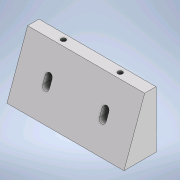
# Autodesk Inventor part: Motorhalterung_BT2.1
Saved by Autodesk Inventor 2020.1 (Build 241239000, 239)
## iProperties
Created: 2020-08-18
Part Number: Motorhalterung_BT2.1
Material: Generisch
Document SubType Name: Modeling
Designer: s5chfeis
Density: 1 g/cm^3
Appearance: Vorgabe
Author: s5chfeis
Autodesk Inventor part; units mm, degrees
ref_plane "YZ Plane" through (0, 0, 0) normal (1, 0, 0) x (0, 1, 0)
ref_plane "XZ Plane" through (0, 0, 0) normal (0, 1, 0) x (-1, 0, 0)
ref_plane "XY Plane" through (0, 0, 0) normal (0, 0, 1) x (1, 0, 0)
sketch "Skizze1" plane through (0, 0, 0) normal (0, 1, 0) x (-1, 0, 0)
  line L0 (0, 0) -> (-206, 0)
  line L1 (-206, 0) -> (-206, -20)
  line L2 (-206, -20) -> (0, -20)
  line L3 (0, -20) -> (0, 0)
  dimension "d0" = 206
  dimension "d1" = 20
  constraints: 8 end point, 2 parallel, 1 horizontal, 1 perpendicular
  measures "d0" distance of L2.end L1.end
  measures "d1" distance of L1.end L0.end
extrude "Extrusion1" add sketch "Skizze1" against normal blind 100
sketch "Skizze2" plane through (0, 0, 0) normal (0, 1, 0) x (1, 0, 0)
  line L0 (0, 0) -> (0, 10) construction
  line L1 (0, 10) -> (206, 10) construction
  line L2 (0, 10) -> (103, 10) construction
  line L3 (103, 10) -> (53, 10) construction
  line L4 (53, 10) -> (153, 10) construction
  dimension "d4" = 10
  dimension "d5" = 206
  dimension "d6" = 90
  dimension "d7" = 103
  dimension "d8" = 50
  dimension "d9" = 100
  constraints: 10 end point, 2 coincident, 2 point on line, 1 midpoint, 1 perpendicular, 1 vertical
  measures "d4" distance of L0.start L0.end
  measures "d5" distance of L0.end L1.end
  measures "d6" angle of L0 L1
  measures "d7" distance of L0.end L2.end
  measures "d8" distance of L2.end L3.end
  measures "d9" distance of L3.end L4.end
hole "Bohrung1" at (153, 0, -10) at (53, 0, -10) direction (0, -1, 0) diameter 8.376 depth 27.3 tip angle 118 thread size "M10x1.5" class "6H" standard "ISO Metric profile"
sketch "Skizze3" plane through (206, 0, 0) normal (1, 0, 0) x (0, 0, -1)
  line L0 (0, 0) -> (-41.0424, -112.7631)
  line L1 (0, 0) -> (120, 0) construction
  line L2 (0, 0) -> (0, -100) projected
  line L3 (0, -100) -> (-50, -100)
  line L4 (0, -100) -> (50, -100) construction
  point P0 (-36.397, -100)
  dimension "d17" = 120
  dimension "d18" = 110
  dimension "d19" = 50
  dimension "d20" = 180
  constraints: 8 end point, 3 horizontal, 2 equal length
  measures "d17" distance of L0.start L0.end
  measures "d18" angle of L0 L1
  measures "d19" distance of L2.end L3.end
  measures "d20" angle of L3 L4
extrude "Extrusion2" add sketch "Skizze3" against normal blind 206
sketch "Skizze4" plane through (206, 0, -20) normal (0, 0, -1) x (-1, 0, 0)
  line L0 (206, 0) -> (103, 0) construction
  line L1 (206, 0) -> (309, 0) construction
  line L2 (103, 0) -> (153, 0) construction
  line L3 (0, 0) -> (206, 0) construction
  line L4 (153, 0) -> (53, 0) construction
  line L5 (53, 0) -> (53, -50) construction
  line L6 (53, 0) -> (103, 0) construction
  line L7 (153, 0) -> (153, -50) construction
  line L8 (153, 0) -> (203, 0) construction
  line L9 (53, -50) -> (59, -50)
  line L10 (59, -50) -> (59, -44)
  arc A0 (59, -44) -> (47, -44) centre (53, -44) ccw
  line L11 (53, -44) -> (47, -44) construction
  line L12 (53, -44) -> (59, -44) construction
  line L13 (47, -44) -> (47, -50)
  line L14 (47, -50) -> (59, -50) construction
  line L15 (53, -100) -> (53, -50) construction
  line L16 (59, -50) -> (59, -56)
  arc A1 (47, -56) -> (59, -56) centre (53, -56) ccw
  line L17 (53, -56) -> (47, -56) construction
  line L18 (53, -56) -> (59, -56) construction
  line L19 (47, -56) -> (47, -50)
  line L20 (103, 0) -> (103, -100) construction
  line L21 (103, 0) -> (203, 0) construction
  line L22 (153, -50) -> (147, -50)
  line L23 (147, -50) -> (147, -44)
  arc A2 (159, -44) -> (147, -44) centre (153, -44) ccw
  line L24 (153, -44) -> (159, -44) construction
  line L25 (153, -44) -> (147, -44) construction
  line L26 (159, -44) -> (159, -50)
  line L27 (159, -50) -> (147, -50) construction
  line L28 (147, -50) -> (147, -56)
  line L29 (153, -56) -> (147, -56) construction
  line L30 (153, -56) -> (159, -56) construction
  line L31 (159, -56) -> (159, -50)
  arc A3 (147, -56) -> (159, -56) centre (153, -56) ccw
  dimension "d23" = 103
  dimension "d24" = 180
  dimension "d25" = 50
  dimension "d26" = 100
  dimension "d27" = 0
  dimension "d28" = 50
  dimension "d29" = 90
  dimension "d30" = 50
  dimension "d31" = 90
  dimension "d32" = 6
  dimension "d33" = 6
  dimension "d34" = 180
  dimension "d35" = 100
  dimension "d36" = 90
  constraints: 62 end point, 15 symmetric about line, 8 point on circle, 7 horizontal, 4 centre point, 4 equal length, 3 perpendicular, 3 point on line, 2 vertical, 1 collinear, 3 other
  measures "d23" distance of L0.start L0.end
  measures "d24" angle of L0 L1
  measures "d25" distance of L0.end L2.end
  measures "d26" distance of L2.end L4.end
  measures "d27" distance between parallel lines of L4 L2
  measures "d28" distance of L4.end L5.end
  measures "d29" angle of L5 L6
  measures "d30" distance of L2.end L7.end
  measures "d31" angle of L7 L8
  measures "d32" distance of L5.end L9.end
  measures "d33" distance of L9.end L10.end
  measures "d34" angle of L12 L11
  measures "d35" distance of L6.end L20.end
  measures "d36" angle of L20 L21
extrude "Extrusion3" cut sketch "Skizze4" against normal blind 100
sketch "Skizze5" plane through (206, 0, -20) normal (0, 0, -1) x (-1, 0, 0)
  line L0 (206, 0) -> (0, 0) projected
  line L1 (103, 0) -> (103, -100)
  line L2 (206, -100) -> (0, -100) projected
  line L3 (0, 0) -> (0, -100) projected
  line L4 (0, -50) -> (206, -50)
  line L5 (206, 0) -> (206, -100) projected
  line L6 (103, -50) -> (68, -50)
  line L7 (68, -50) -> (68, -30)
  line L8 (68, -30) -> (103, -30)
  line L9 (103, -30) -> (103, -50)
  line L10 (103, -50) -> (138, -50)
  line L11 (138, -50) -> (138, -30)
  line L12 (138, -30) -> (103, -30)
  line L13 (68, -50) -> (68, -70)
  line L14 (68, -70) -> (103, -70)
  line L15 (103, -70) -> (103, -50)
  line L16 (138, -50) -> (138, -70)
  line L17 (138, -70) -> (103, -70)
  dimension "d39" = 35
  dimension "d40" = 20
  constraints: 28 end point, 5 midpoint, 5 symmetric about line, 2 parallel, 1 horizontal, 1 perpendicular
  measures "d39" distance of L7.end L8.end
  measures "d40" distance of L6.end L7.end
extrude "Extrusion4" add sketch "Skizze5" along normal blind 30 contours L12 L11 L4 L1 | L1 L4 L7 L8 | L16 L17 L1 L4 | L1 L14 L13 L4
sketch "Skizze6" plane through (68, -30, -20) normal (0, 1, 0) x (1, 0, 0)
  line L0 (70, 30) -> (0, 30) projected
  circle A0 centre (35, 30) radius 17.5
  point P0 (-68, -20)
  dimension "d43" = 35
  constraints: 1 centre point, 1 midpoint
  measures "d43" diameter of A0
extrude "Extrusion5" cut sketch "Skizze6" against normal blind 40
sketch "Skizze7" plane through (68, -30, -20) normal (0, 1, 0) x (1, 0, 0)
  arc A0 (17.5, 30) -> (52.5, 30) centre (35, 30) ccw projected
  line L0 (35, 12.5) -> (35, 13.5)
  line L1 (35, 12.5) -> (36, 12.5) construction
  line L2 (35, 13.5) -> (45, 13.5)
  line L3 (45, 13.5) -> (25, 13.5)
  point P0 (-68, -20)
  point P1 (35, 13.5)
  point P2 (29.169, 13.5)
  point P3 (40.831, 13.5)
  dimension "d46" = 1
  dimension "d47" = 90
  dimension "d48" = 10
  dimension "d49" = 90
  dimension "d50" = 20
  dimension "d51" = 0
  constraints: 8 end point, 2 perpendicular, 1 collinear, 1 horizontal, 1 point on circle, 1 vertical
  measures "d46" distance of L0.start L0.end
  measures "d47" angle of L1 L0
  measures "d48" distance of L0.end L2.end
  measures "d49" angle of L0 L2
  measures "d50" distance of L2.end L3.end
  measures "d51" distance between parallel lines of L3 L2
extrude "Extrusion6" add sketch "Skizze7" against normal blind 40
sketch "Skizze8" plane through (206, 0, -50) normal (0, 0, -1) x (-1, 0, 0)
  line L0 (68, -30) -> (138, -30) construction
  line L1 (85.5, -70) -> (85.5, -30) construction
  line L2 (68, -30) -> (85.5, -70) construction
  line L3 (138, -70) -> (68, -70) construction
  line L4 (68, -70) -> (85.5, -30) construction
  line L5 (103, -30) -> (103, -70) construction
  line L6 (120.5, -70) -> (120.5, -30) construction
  line L7 (138, -30) -> (120.5, -70) construction
  line L8 (138, -70) -> (120.5, -30) construction
  point P0 (206, 0)
  point P1 (76.75, -50)
  point P2 (129.25, -50)
  constraints: 12 end point, 3 midpoint, 3 symmetric about line
hole "Bohrung2" at (129.25, -50, -50) at (76.75, -50, -50) direction (0, 0, 1) diameter 8.376 depth 27.3 tip angle 118 thread size "M10x1.5" class "6H" standard "ISO Metric profile"
